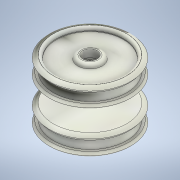
# Autodesk Inventor part: kolo_vetsi
Saved by Autodesk Inventor 2022 (Build 260153000, 153)
## iProperties
Created: 2022-11-21
Part Number: kolo_vetsi
Material: Generic
Document SubType Name: Modeling
Designer: matys
Density: 1 g/cm^3
Appearance: Default
Author: matys
Autodesk Inventor part; units mm, degrees
ref_plane "YZ Plane" through (0, 0, 0) normal (1, 0, 0) x (0, 1, 0)
ref_plane "XZ Plane" through (0, 0, 0) normal (0, 1, 0) x (-1, 0, 0)
ref_plane "XY Plane" through (0, 0, 0) normal (0, 0, 1) x (1, 0, 0)
sketch "Sketch1" plane through (0, 0, 0) normal (0, 1, 0) x (-1, 0, 0)
  line L0 (0, 0) -> (17, 0)
  circle A0 centre (0, 0) radius 17
  line L1 (0, 0) -> (0, -4)
  dimension "d0" = 17
  dimension "d1" = 4
  constraints: 4 end point, 1 coincident, 1 horizontal, 1 horizontal alignment, 1 vertical, 2 other
  measures "d0" distance of L0.start L0.end
  measures "d1" distance of L1.start L1.end
extrude "Extrusion1" add sketch "Sketch1" along normal blind 8
sketch "Sketch2" plane through (0, 8, 0) normal (0, 1, 0) x (1, 0, 0)
  circle A0 centre (0, 0) radius 2
  dimension "d4" = 4
  constraints: 1 centre point, 1 coincident
  measures "d4" diameter of A0
extrude "Extrusion2" add sketch "Sketch2" along normal blind 9
sketch "Sketch3" plane through (0, 17, 0) normal (0, 1, 0) x (1, 0, 0)
  circle A0 centre (0, 0) radius 17
  constraints: 1 centre point, 1 coincident
extrude "Extrusion3" add sketch "Sketch3" along normal blind 2
sketch "Sketch4" plane through (0, 19, 0) normal (0, 1, 0) x (1, 0, 0)
  circle A0 centre (0, 0) radius 1.1
  dimension "d9" = 2.2
  constraints: 1 centre point, 1 coincident
  measures "d9" diameter of A0
extrude "Extrusion4" cut sketch "Sketch4" against normal through all
sketch "Sketch5" plane through (0, 19, 0) normal (0, 1, 0) x (1, 0, 0)
  circle A0 centre (0, 0) radius 1.1 projected
  line L0 (0, 0) -> (-15, 0)
  circle A1 centre (0, 0) radius 15
  dimension "d12" = 15
  constraints: 2 end point, 1 coincident, 1 horizontal, 1 horizontal alignment, 2 other
  measures "d12" distance of L0.start L0.end
extrude "Extrusion5" add sketch "Sketch5" along normal blind 4
sketch "Sketch6" plane through (0, 23, 0) normal (0, 1, 0) x (1, 0, 0)
  circle A0 centre (0, 0) radius 1.1 projected
  circle A1 centre (0, 0) radius 17
  constraints: 1 centre point, 1 coincident
extrude "Extrusion6" add sketch "Sketch6" along normal blind 2
fillet "Fillet1" radius 2 2 edges at (-17, 25, 0) (-17, 17, 0)
chamfer "Chamfer2" distance 1 angle 45 4 edges at (-17, 19, 0) (-17, 18.9995, 0) (-17, 23.0005, 0) (-17, 23, 0)
sketch "Sketch7" plane through (0, 0, 0) normal (0, 0, 1) x (1, 0, 0)
  line L0 (0, 0) -> (0, 25)
  line L1 (-15, 25) -> (15, 25) projected
  line L2 (0, 12.5) -> (17, 12.5)
  line L3 (17, 12.5) -> (17, 0)
  line L4 (17, 0) -> (-17, 0) projected
  line L5 (17, 0) -> (-17, 0)
  line L6 (-17, 0) -> (-17, 12.5)
  line L7 (-17, 12.5) -> (17, 12.5)
  dimension "d24" = 17
  constraints: 12 end point, 4 perpendicular, 2 midpoint, 1 horizontal, 1 point on line
  measures "d24" distance of L2.start L2.end
extrude "Extrusion7" cut sketch "Sketch7" along normal through all both and the other way through all
mirror "Mirror1" about plane through (17, 12.5, 0) normal (0, -1, 0)
sketch "Sketch8" plane through (0, 25, 0) normal (0, 1, 0) x (1, 0, 0)
  circle A0 centre (0, 0) radius 2 projected
  circle A1 centre (0, 0) radius 1.1 projected
  circle A2 centre (0, 0) radius 13.75
  circle A3 centre (0, 0) radius 3
  circle A4 centre (0, 0) radius 5
  dimension "d30" = 27.5
  dimension "d32" = 6
  dimension "d33" = 10
  constraints: 3 centre point, 3 coincident
  measures "d30" diameter of A2
  measures "d32" diameter of A3
  measures "d33" diameter of A4
extrude "Extrusion8" cut sketch "Sketch8" against normal blind 1.5 contours A0 | A1 | A2 | A3
fillet "Fillet2" radius 1.2 1 edges at (-13.75, 25, 0)
fillet "Fillet3" radius 1.5 1 edges at (-5, 25, 0)
sketch "Sketch9" plane through (0, 25, 0) normal (0, 1, 0) x (1, 0, 0)
  circle A0 centre (0, 0) radius 3
  dimension "d45" = 6
  constraints: 1 centre point, 1 coincident
  measures "d45" diameter of A0
extrude "Extrusion9" cut sketch "Sketch9" against normal blind 3.2
sketch "Sketch10" plane through (0, 21.8, 0) normal (0, 1, 0) x (1, 0, 0)
  circle A0 centre (0, 0) radius 2
  dimension "d37" = 4
  constraints: 1 centre point, 1 coincident
  measures "d37" diameter of A0
extrude "Extrusion10" cut sketch "Sketch10" against normal blind 5
sketch "Sketch11" plane through (0, 8, 0) normal (0, 1, 0) x (1, 0, 0)
  circle A0 centre (0, 0) radius 2
  circle A1 centre (0, 0) radius 1.1 projected
  circle A2 centre (0, 0) radius 2.6
  dimension "d40" = 5.2
  constraints: 2 centre point, 2 coincident
  measures "d40" diameter of A2
extrude "Extrusion11" add sketch "Sketch11" along normal blind 9 contours A2
sketch "Sketch12" plane through (0, 16.8, 0) normal (0, 1, 0) x (1, 0, 0)
  circle A0 centre (0, 0) radius 2
  circle A1 centre (0, 0) radius 2 projected
  line L0 (-2, 0) -> (0, 2)
  line L1 (0, 2) -> (2, 0)
  line L2 (2, 0) -> (0, -2)
  line L3 (0, -2) -> (-2, 0)
  constraints: 8 end point, 2 parallel, 2 point on circle, 1 centre point, 1 coincident, 1 perpendicular
extrude "Extrusion12" cut sketch "Sketch12" against normal blind 6 contours L2 L3 L0 L1
body "Solid1"
